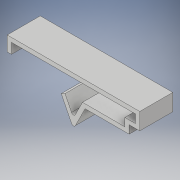
# Autodesk Inventor part: Wood Rail Selector Conductor
Saved by Autodesk Inventor 2018 (Build 220112000, 112)
## iProperties
Created: 2017-12-04
Part Number: Wood Rail Selector Conductor
Material: Generic
Document SubType Name: Modeling
Designer: Andrew
Density: 1 g/cm^3
Appearance: Default
Author: Andrew
Autodesk Inventor part; units mm, degrees
ref_plane "YZ Plane" through (0, 0, 0) normal (1, 0, 0) x (0, 1, 0)
ref_plane "XZ Plane" through (0, 0, 0) normal (0, 1, 0) x (-1, 0, 0)
sketch "Sketch1" plane through (0, 0, 0) normal (0, 0, 1) x (1, 0, 0)
  line L0 (-9.8524, 0) -> (9.8524, 0)
  line L1 (9.8524, 0) -> (9.8524, -1.9248)
  line L2 (9.8524, -1.9248) -> (8.2268, -1.9248)
  line L3 (8.2268, -1.9248) -> (8.2268, -3.175)
  line L4 (8.2268, -3.175) -> (1.5875, -3.175)
  line L5 (1.5875, -3.175) -> (0, -6.35)
  line L6 (0, -6.35) -> (-1.5875, -3.175)
  line L7 (-9.8524, 0) -> (-9.8524, -1.9248)
  line L8 (0, 1.27) -> (0, -7.62) projected
  point P0 (0, 0)
  dimension "d0" = 19.7048
  dimension "d2" = 1.9248
  dimension "d3" = 6.35
  dimension "d4" = 3.175
  dimension "d5" = 1.6256
  dimension "d6" = 3.175
  constraints: 16 end point, 4 perpendicular, 2 point on line, 1 horizontal, 1 midpoint, 1 vertical, 2 other
  measures "d0" distance of L0.start L0.end
  measures "d2" distance of L0.end L1.end
  measures "d3" distance from line of L5.end L0
  measures "d4" distance from line of L5.end L4
  measures "d5" distance of L1.end L2.end
  measures "d6" distance of L4.end L6.end
derived "Conductive Rail.ipt"
ref_plane "Work Plane1" through (-9.8524, -1.9248, 0) normal (0, -1, 0) x (1, 0, 0)
sketch "Sketch2" plane through (-9.8524, -1.9248, 0) normal (0, -1, 0) x (1, 0, 0)
  line L0 (0.3274, 2.54) -> (-0.3274, 2.54)
  line L1 (-0.3274, 2.54) -> (-0.3274, -2.54)
  line L2 (-0.3274, -2.54) -> (0.3274, -2.54)
  line L3 (0.3274, -2.54) -> (0.3274, 2.54)
  line L4 (0.3274, 2.54) -> (-0.3274, -2.54) construction
  line L5 (-0.3274, 2.54) -> (0.3274, -2.54) construction
  point P0 (9.8524, 0)
  point P1 (0, 0)
  point P2 (0, 0)
  point P3 (0, 0)
  dimension "d7" = 5.08
  dimension "d8" = 0.6548
  constraints: 12 end point, 2 midpoint, 2 parallel, 1 horizontal, 1 perpendicular
  measures "d7" distance of L0.end L1.end
  measures "d8" distance of L0.start L0.end
sweep "Sweep1" add profiles "Sketch2" path "Sketch1" path curves L7 L0 L1 L2 L3 L4 L5 L6
fillet "Fillet1" radius 0.3274 2 edges at (0, -7.0821, 0) (0, -5.6179, 0)
equation "\"d7\" = springSteelWidth"
equation "\"d8\" = springSteelThickness"
equation "\"d11\" = 0.5 * springSteelThickness"
equation "\"springSteelWidth\" = 5.08"
equation "\"springSteelThickness\" = 0.6548"
body "Solid1"
